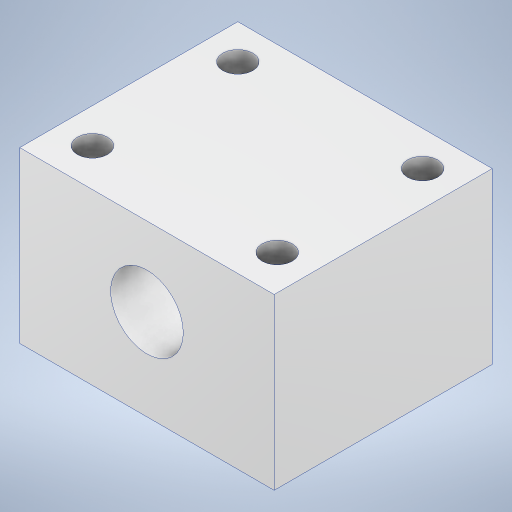
# Autodesk Inventor part: Linear Bearing Slide Unit 12mm (Technobots)
Saved by Autodesk Inventor 2023.2 (Build 272271000, 271)
## iProperties
Created: 2023-01-31
Part Number: Linear Bearing Slide Unit 12mm (Technobots)
Material: Aluminum 6061
Document SubType Name: Modeling
Designer: dmargari
Density: 2.7 g/cm^3
Appearance: Aluminum - Flat
Author: dmargari
Autodesk Inventor part; units mm, degrees
ref_plane "YZ Plane" through (0, 0, 0) normal (1, 0, 0) x (0, 1, 0)
ref_plane "XZ Plane" through (0, 0, 0) normal (0, 1, 0) x (-1, 0, 0)
ref_plane "XY Plane" through (0, 0, 0) normal (0, 0, 1) x (1, 0, 0)
sketch "Sketch1" plane through (0, 0, 0) normal (0, 0, 1) x (1, 0, 0)
  line L0 (4.3397, 2.4857) -> (46.3397, 2.4857)
  line L1 (4.3397, 2.4857) -> (46.3397, 2.4857) construction
  line L2 (46.3397, 2.4857) -> (46.3397, -25.5143)
  line L3 (46.3397, 2.4857) -> (74.3397, 2.4857) construction
  line L4 (46.3397, -25.5143) -> (4.3397, -25.5143)
  line L5 (4.3397, -25.5143) -> (4.3397, 2.4857)
  circle A0 centre (25.3397, -10.5143) radius 6
  point P0 (0, 0)
  point P1 (25.3397, -25.5143)
  dimension "d0" = 42
  dimension "d2" = 28
  dimension "d3" = 90
  dimension "d4" = 12
  dimension "d5" = 15
  constraints: 12 end point, 3 horizontal, 2 equal length, 2 perpendicular, 1 centre point, 1 midpoint, 1 vertical
  measures "d0" distance of L0.start L0.end
  measures "d2" distance of L1.end L2.end
  measures "d3" angle of L2 L3
  measures "d4" diameter of A0
  measures "d5" distance of point (25.34, -25.514) A0.centre
extrude "Extrusion1" add sketch "Sketch1" along normal mid plane 36
sketch "Sketch2" plane through (4.3397, 2.4857, 18) normal (0, 1, 0) x (1, 0, 0)
  line L0 (0, 36) -> (42, 36) construction
  line L1 (0, 0) -> (42, 0) construction
  line L2 (0, 36) -> (0, 0) construction
  line L3 (42, 0) -> (0, 0) construction
  line L4 (42, 36) -> (42, 0) construction
  line L5 (0, 36) -> (42, 36) construction
  line L6 (5.75, 36) -> (5.75, 0) construction
  line L7 (0, 36) -> (0, 0) construction
  line L8 (0, 30.25) -> (42, 30.25) construction
  line L9 (42, 36) -> (42, 0) construction
  circle A0 centre (5.75, 30.25) radius 2.5
  line L10 (0, 18.25) -> (42, 18.25) construction
  line L11 (42, 36) -> (42, 0) construction
  circle A1 centre (5.75, 6.25) radius 2.5
  line L12 (42, 0) -> (0, 0) construction
  line L13 (21, 0) -> (21, 36) construction
  circle A2 centre (36.25, 30.25) radius 2.5
  circle A3 centre (36.25, 6.25) radius 2.5
  point P0 (-4.3397, 18)
  dimension "d8" = 5.75
  dimension "d9" = 5.75
  dimension "d10" = 5
  dimension "d11" = 12
  dimension "d12" = 15.25
  constraints: 8 end point, 8 point on line, 4 centre point, 3 perpendicular, 3 symmetric about line, 2 midpoint, 1 horizontal, 3 other
  measures "d8" distance between parallel lines of L2 L6
  measures "d9" distance between parallel lines of L0 L8
  measures "d10" diameter of A0
  measures "d11" distance between parallel lines of L8 L10
  measures "d12" distance between parallel lines of L6 L13
extrude "Extrusion2" cut sketch "Sketch2" against normal through all
body "Solid1"
